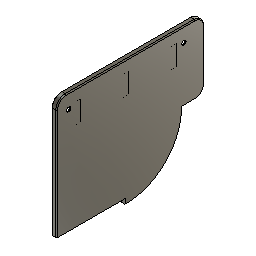
Reduzierplatten_Halter (Autodesk Fusion 360 design; units mm, degrees)
Autodesk Fusion 360 part; units mm, degrees
sketch "Sketch1" plane through (0, 0, 0) normal (1, 0, 0) x (0, 1, 0)
  arc A0 (-1.3693, -52.3821) -> (52.3821, 1.3693) centre (0, 0) ccw
  arc A1 (-1.3693, -52.3821) -> (-6.5, -57.3804) centre (-1.5, -57.3804) ccw
  arc A2 (57.3804, 6.5) -> (52.3821, 1.3693) centre (57.3804, 1.5) ccw
  line L0 (-2.4, 39.5) -> (2.4, 39.5)
  line L1 (2.4, 39.5) -> (2.4, 60.5)
  line L2 (2.4, 60.5) -> (-2.4, 60.5)
  line L3 (-2.4, 60.5) -> (-2.4, 39.5)
  line L4 (-2.4, 39.5) -> (2.4, 60.5) construction
  line L5 (2.4, 39.5) -> (-2.4, 60.5) construction
  line L6 (-6.5, -57.3804) -> (-6.5, -71.5)
  line L7 (57.3804, 6.5) -> (71.5, 6.5)
  line L8 (-66.5, -71.5) -> (-66.5, 62.5)
  line L9 (-62.5, 66.5) -> (71.5, 66.5)
  line L10 (-10.5, -75.5) -> (-62.5, -75.5)
  line L11 (75.5, 62.5) -> (75.5, 10.5)
  arc A3 (-10.5, -75.5) -> (-6.5, -71.5) centre (-10.5, -71.5) ccw
  arc A4 (-66.5, -71.5) -> (-62.5, -75.5) centre (-62.5, -71.5) ccw
  arc A5 (-62.5, 66.5) -> (-66.5, 62.5) centre (-62.5, 62.5) ccw
  arc A6 (75.5, 62.5) -> (71.5, 66.5) centre (71.5, 62.5) ccw
  arc A7 (71.5, 6.5) -> (75.5, 10.5) centre (71.5, 10.5) ccw
  arc A8 (-62.5, 72.5) -> (-72.5, 62.5) centre (-62.5, 62.5) ccw
  line L12 (-72.5, -71.5) -> (-72.5, 62.5)
  arc A9 (-72.5, -71.5) -> (-62.5, -81.5) centre (-62.5, -71.5) ccw
  line L13 (-10.5, -81.5) -> (-62.5, -81.5)
  arc A10 (-10.5, -81.5) -> (-0.5, -71.5) centre (-10.5, -71.5) ccw
  line L14 (-0.5, -58.3979) -> (-0.5, -71.5)
  arc A11 (-0.5, -58.3979) -> (58.3979, 0.5) centre (0, 0) ccw
  line L15 (58.3979, 0.5) -> (71.5, 0.5)
  arc A12 (71.5, 0.5) -> (81.5, 10.5) centre (71.5, 10.5) ccw
  line L16 (81.5, 62.5) -> (81.5, 10.5)
  arc A13 (81.5, 62.5) -> (71.5, 72.5) centre (71.5, 62.5) ccw
  line L17 (-62.5, 72.5) -> (71.5, 72.5)
  line L18 (-72.5, -52.4) -> (0, -52.4)
  line L19 (-0.5, -58.3979) -> (-0.5, -52.4)
  line L20 (60, 57.5) -> (-60, 57.5) construction
  point P0 (51.6797, 8.6582)
  point P1 (0, 50)
  point P2 (-66.5, -75.5)
  point P3 (-66.5, 66.5)
  point P4 (0, 57.5)
  dimension "d6" = 52.4
  dimension "d12" = 5
  dimension "d36" = 6.5
  dimension "d37" = 6.5
  dimension "d39" = 142
  dimension "d40" = 60
  dimension "d41" = 4
  dimension "d42" = 60
  dimension "d43" = -6
  dimension "d44" = 50
  dimension "d45" = 21
  dimension "d46" = 4.8
  dimension "d51" = 120
  dimension "d52" = 15
  constraint coincident A0.centre A11.centre
  constraint tangent A0 A1
  constraint coincident P0 A0
  constraint tangent A0 A2
  constraint equal A1 A2
  constraint horizontal L0
  constraint perpendicular L0 L1
  constraint parallel L0 L2
  constraint parallel L1 L3
  constraint coincident L4 P1
  constraint coincident L5 P1
  constraint tangent A1 L6
  constraint tangent A2 L7
  constraint horizontal L7
  constraint coincident A0 L18.end
  constraint vertical L6
  constraint perpendicular L7 L11
  constraint vertical L8
  constraint horizontal L10
  constraint horizontal L9
  constraint tangent L6 A3
  constraint tangent L10 A3
  constraint coincident P2 L8
  constraint coincident P2 L10
  constraint tangent L8 A4
  constraint tangent L10 A4
  constraint equal A3 A4
  constraint coincident P3 L8
  constraint coincident P3 L9
  constraint tangent L8 A5
  constraint tangent L9 A5
  constraint equal A3 A5
  constraint tangent L9 A6
  constraint tangent L11 A6
  constraint equal A3 A6
  constraint tangent L7 A7
  constraint tangent L11 A7
  constraint equal A3 A7
  constraint equal L6 L7
  constraint coincident L12 L18.start
  constraint horizontal L18
  constraint tangent A0 L18
  constraint vertical P1 A0.centre
  constraint coincident L18 L19.end
  constraint perpendicular L18 L19
  constraint horizontal L20
  constraint midpoint L20 P4
  constraint vertical A0.centre P4
  measures "d6" radius of A0
  measures "d12" radius of A2
  measures "d36" distance of A0.centre L7
  measures "d37" distance of A0.centre L6
  measures "d39" vertical distance of P2 P3
  measures "d40" distance of L6 L8
  measures "d41" radius of A3
  measures "d42" distance of L7 L9
  measures "d44" distance of A0.centre P1
  measures "d45" distance of L0.start L2.end
  measures "d46" distance of L1.end L2.end
  measures "d51" distance of L20.start L20.end
  measures "d52" distance of L17 L20
extrude "Extrude1" add sketch "Sketch1" along normal blind 5.5 contours A0 A1 A2 L7 L8 L9 L11 A5 A6 A7 L18 | A0 A2 L7 L8 L9 L11 A5 A6 A7 A8 L12 A11 L15 A12 L16 A13 L17 L18 L19 | L0 L1 L2 L3
extrude "Extrude2" cut sketch "Sketch1" along normal blind 2.5 contours A0 A1 A2 L7 L8 L9 L11 A5 A6 A7 L18 | A1 L6 L8 L10 A3 A4 L18 | L0 L1 L2 L3
extrude "Extrude3" cut sketch "Sketch1" along normal blind 2.4 from surface at 2.5 contours L0 L1 L2 L3
pattern_linear "R-Pattern1" count 3 spacing 50 along (0, 1, 0) both ways of "Extrude3"
hole "Hole1" at (0, 60, 57.5) at (0, -60, 57.5) direction (1, 0, 0) diameter 4.5 end through all countersink diameter 14 countersink angle 90
chamfer "Chamfer2" distance 1 angle 45 16 edges at (5.5, -72.5, 5.05) (5.5, -69.5711, 69.5711) (5.5, 4.5, 72.5) (5.5, 78.5711, 69.5711) (5.5, 81.5, 36.5) (5.5, 78.5711, 3.4289) (5.5, 64.9489, 0.5) (5.5, 41.295, -41.295) (0, 64.9489, 0.5) (0, 78.5711, 3.4289) (0, 81.5, 36.5) (0, 78.5711, 69.5711) (0, 4.5, 72.5) (0, -69.5711, 69.5711) (0, -72.5, 5.05) (0, 41.295, -41.295)
chamfer "Chamfer2" distance 0.4 angle 45 11 edges at (0, -66.5, 61.299) (0, -65.3284, 65.3284) (0, 4.5, 66.5) (0, 74.3284, 65.3284) (0, 75.5, 36.5) (0, 74.3284, 7.6716) (0, 64.4402, 6.5) (0, 53.799, 4.989) (0, 37.5334, -36.5651) (0, -0.25, -52.4) (0, -66.5, 1.251)
